budvar_holder (Autodesk Fusion 360 design; units mm, degrees)
Autodesk Fusion 360 part; units mm, degrees
sketch "Sketch1" plane through (0, 0, 0) normal (0, 1, 0) x (1, 0, 0)
  circle A0 centre (-139, -97.5) radius 1.5
  circle A1 centre (139, -97.5) radius 1.5
  circle A2 centre (139, 97.5) radius 1.5
  circle A3 centre (-139, 97.5) radius 1.5
  line L0 (139, -97.5) -> (139, 97.5) construction
  line L1 (139, 97.5) -> (-139, 97.5) construction
  line L2 (-139, 97.5) -> (-139, -97.5) construction
  line L3 (-139, -97.5) -> (139, -97.5) construction
  line L4 (0, -97.5) -> (0, 97.5) construction
  line L5 (139, 0) -> (-139, 0) construction
  circle A4 centre (-139, -97.5) radius 4
  circle A5 centre (-139, 97.5) radius 4
  circle A6 centre (139, 97.5) radius 4
  circle A7 centre (139, -97.5) radius 4
  line L6 (-143, -97.5) -> (-135, -97.5)
  line L7 (-135, -97.5) -> (-135, 97.5)
  line L8 (-135, 97.5) -> (-143, 97.5)
  line L9 (-143, 97.5) -> (-143, -97.5)
  line L10 (143, -97.5) -> (135, -97.5)
  line L11 (135, -97.5) -> (135, 97.5)
  line L12 (135, 97.5) -> (143, 97.5)
  line L13 (143, 97.5) -> (143, -97.5)
  line L14 (-143, -5) -> (143, -5)
  line L15 (143, -5) -> (143, 5)
  line L16 (143, 5) -> (-143, 5)
  line L17 (-143, 5) -> (-143, -5)
  line L18 (-35, -5) -> (-136.2569, -100.4112)
  line L19 (-46.6654, -5) -> (-141.7431, -94.5888)
  line L20 (-136.2569, -100.4112) -> (-141.7431, -94.5888)
  line L21 (35, -5) -> (136.2569, -100.4112)
  line L22 (46.6654, -5) -> (141.7431, -94.5888)
  line L23 (136.2569, -100.4112) -> (141.7431, -94.5888)
  line L24 (-35, 5) -> (-136.2569, 100.4112)
  line L25 (-46.6654, 5) -> (-141.7431, 94.5888)
  line L26 (46.6654, 5) -> (141.7431, 94.5888)
  line L27 (35, 5) -> (136.2569, 100.4112)
  line L28 (136.2569, 100.4112) -> (141.7431, 94.5888)
  line L29 (-136.2569, 100.4112) -> (-141.7431, 94.5888)
  circle A8 centre (-14, 0) radius 1.25
  circle A9 centre (14, 0) radius 1.25
  dimension "d1" = 3
  dimension "d2" = 3
  dimension "d3" = 3
  dimension "d4" = 3
  dimension "d5" = 278
  dimension "d6" = 195
  dimension "d7" = 8
  dimension "d8" = 8
  dimension "d9" = 8
  dimension "d10" = 8
  dimension "d11" = 5
  dimension "d12" = 5
  dimension "d13" = 35
  dimension "d14" = 2.5
  dimension "d15" = 2.5
  dimension "d16" = 14
  dimension "d17" = 14
  constraint coincident A1.centre L0.start
  constraint coincident A2.centre L0.end
  constraint vertical L0
  constraint coincident A3.centre L1.end
  constraint perpendicular L0 L1
  constraint coincident A0.centre L2.end
  constraint perpendicular L1 L2
  constraint perpendicular L0 L3
  constraint midpoint L3 L4.start
  constraint midpoint L1 L4.end
  constraint midpoint L0 L5.start
  constraint midpoint L2 L5.end
  constraint midpoint origin L4
  constraint concentric A0 A4
  constraint concentric A2 A6
  constraint concentric A1 A7
  constraint horizontal L6
  constraint vertical L7
  constraint horizontal L8
  constraint vertical L9
  constraint coincident A5 L7.end
  constraint coincident L1 L7.end
  constraint coincident A4 L6.start
  constraint horizontal L10
  constraint vertical L11
  constraint horizontal L12
  constraint vertical L13
  constraint coincident A6 L11.end
  constraint coincident L1 L11.end
  constraint coincident A7 L10.start
  constraint midpoint A0.centre L6
  constraint midpoint A1.centre L10
  constraint horizontal L14
  constraint vertical L15
  constraint horizontal L16
  constraint vertical L17
  constraint coincident L13 L15.end
  constraint coincident L9 L14.start
  constraint coincident L14 L18.start
  constraint coincident A4 L18.end
  constraint tangent A4 L18
  constraint coincident L14 L19.start
  constraint coincident A4 L19.end
  constraint parallel L18 L19
  constraint midpoint A0.centre L20
  constraint symmetric L4 L18.start L21.start
  constraint symmetric L4 L18.end L21.end
  constraint symmetric L4 L19.start L22.start
  constraint symmetric L4 L19.end L22.end
  constraint symmetric L5 L18.start L24.start
  constraint symmetric L5 L18.end L24.end
  constraint symmetric L5 L19.start L25.start
  constraint symmetric L5 L19.end L25.end
  constraint symmetric L5 L21.start L27.start
  constraint symmetric L5 L21.end L27.end
  constraint symmetric L5 L22.start L26.start
  constraint symmetric L5 L22.end L26.end
  constraint coincident L5 A8.centre
  constraint coincident L5 A9.centre
  measures "d1" diameter of A0
  measures "d2" diameter of A1
  measures "d3" diameter of A2
  measures "d4" diameter of A3
  measures "d5" distance of A0.centre A1.centre
  measures "d6" distance of A1.centre A2.centre
  measures "d7" diameter of A4
  measures "d8" diameter of A5
  measures "d9" diameter of A7
  measures "d10" diameter of A6
  measures "d11" distance of origin L16
  measures "d12" distance of origin L14
  measures "d13" horizontal distance of origin L18.start
  measures "d14" diameter of A8
  measures "d15" diameter of A9
  measures "d16" distance of origin A9.centre
  measures "d17" distance of origin A8.centre
extrude "Extrude1" add sketch "Sketch1" along normal blind 8.5 contours A0 A4 L6 L20 | A0 A4 L6 L20 | A0 A4 L6 L20 | A0 A4 L6 L20 | A4 L7 L14 L18 L19 | A4 L7 L19 | A4 L7 L9 L14 L19 | L7 L11 L14 L16 | L7 L9 L14 L16 L17 | A7 L11 L14 L21 L22 | A5 L7 L9 L16 L25 | A1 A7 L10 L23 | A1 A7 L10 L23 | A5 L7 L25 | A5 L7 L16 L24 L25 | A3 A5 L8 L29 | A3 A5 L8 L29 | A7 L11 L13 L14 L22 | L11 L13 L14 L15 L16 | A7 L11 L22 | A1 A7 L10 L23 | A1 A7 L10 L23 | A3 A5 L8 L29 | A3 A5 L8 L29 | A6 L11 L13 L16 L26 | A6 L11 L16 L26 L27 | A6 L11 L26 | A2 A6 L12 L28 | A2 A6 L12 L28 | A2 A6 L12 L28 | A2 A6 L12 L28
equation "d2 = d1"
equation "d3 = d2"
equation "d4 = d1"
equation "d8 = d7"
equation "d9 = d7"
equation "d10 = d7"
equation "d12 = d11"
equation "d17 = d16"
